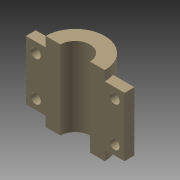
# Autodesk Inventor part: 砂轮架带动曲柄轴盖
Saved by Autodesk Inventor 2015 (Build 190159000, 159)
## iProperties
Created: 2017-05-17
Part Number: 砂轮架带动曲柄轴盖
Material: 常规
Document SubType Name: Modeling
Designer: Administrator
Density: 1 g/cm^3
Appearance: 麦色
Author: Administrator
Autodesk Inventor part; units mm, degrees
ref_plane "YZ Plane" through (0, 0, 0) normal (1, 0, 0) x (0, 1, 0)
ref_plane "XZ Plane" through (0, 0, 0) normal (0, 1, 0) x (-1, 0, 0)
ref_plane "XY Plane" through (0, 0, 0) normal (0, 0, 1) x (1, 0, 0)
sketch "草图1" plane through (0, 0, 0) normal (0, 0, 1) x (1, 0, 0)
  arc A0 (7.5, 0) -> (-7.5, 0) centre (0, 0) ccw
  arc A1 (15, 0) -> (-15, 0) centre (0, 0) ccw
  line L0 (25, 5) -> (25, 0)
  line L1 (-25, 0) -> (-25, 5)
  line L2 (25, 0) -> (7.5, 0)
  line L3 (-7.5, 0) -> (-25, 0)
  line L4 (-25, 5) -> (-5.5902, 5)
  line L5 (5.5902, 5) -> (25, 5)
  line L6 (0, 0) -> (0, -4.0409)
  line L7 (0, 0) -> (2.0046, 0)
  arc A2 (5.5902, 5) -> (-5.5902, 5) centre (0, 0) ccw
  arc A3 (14.1421, 5) -> (-14.1421, 5) centre (0, 0) ccw
  dimension "d0" = 15
  dimension "d1" = 30
  dimension "d2" = 5
  dimension "d3" = 50
  dimension "d4" = 4.0409
  dimension "d5" = 2.0046
  constraints: 16 end point, 12 point on circle, 5 parallel, 4 centre point, 4 point on line, 3 coincident, 3 collinear, 3 horizontal, 2 concentric, 2 perpendicular, 1 vertical, 1 other
  measures "d0" diameter of A0
  measures "d1" diameter of A1
  measures "d2" distance of L0.start L0.end
  measures "d3" distance of L1.end L0.start
  measures "d4" distance of L6.start L6.end
  measures "d5" distance of L6.start L7.end
extrude "拉伸1" add sketch "草图1" along normal blind 40
sketch "草图2" plane through (0, 0, 40) normal (0, 0, 1) x (1, 0, 0)
  line L0 (14.1421, 5) -> (25, 5)
  line L1 (25, 5) -> (14.1421, 5) projected
  line L2 (25, 5) -> (25, 0)
  line L3 (25, 0) -> (15, 0)
  line L4 (7.5, 0) -> (25, 0) projected
  line L5 (-14.1421, 5) -> (-25, 5)
  line L6 (-14.1421, 5) -> (-25, 5) projected
  line L7 (-25, 5) -> (-25, 0)
  line L8 (-25, 0) -> (-15, 0)
  arc A0 (15, 0) -> (14.1421, 5) centre (0, 0) ccw
  arc A1 (-14.1421, 5) -> (-15, 0) centre (0, 0) ccw
  constraints: 12 end point, 4 point on circle, 3 collinear, 3 perpendicular, 2 centre point, 2 coincident, 1 point on line
extrude "拉伸2" cut sketch "草图2" against normal blind 5
pattern_linear "矩形阵列1" count 2 spacing 35 along (0, 0, -1) of "拉伸2"
fillet "圆角1" radius 0.25 2 edges at (14.1421, 5, 20) (-14.1421, 5, 20)
sketch "草图3" plane through (25, 5, 35) normal (0, 1, 0) x (1, 0, 0)
  circle A0 centre (-5, 25) radius 2.5
  circle A1 centre (-5, 5) radius 2.5
  circle A2 centre (-45, 25) radius 2.5
  circle A3 centre (-45, 5) radius 2.5
  line L0 (0, 30) -> (0, 0) projected
  line L1 (0, 30) -> (-10.6822, 30) projected
  line L2 (-10.6822, 0) -> (0, 0) projected
  line L3 (-50, 30) -> (-50, 0) projected
  line L4 (-50, 0) -> (-39.3178, 0) projected
  line L5 (-39.3178, 30) -> (-50, 30) projected
  point P0 (-25, 35)
  dimension "d14" = 5
  dimension "d15" = 5
  dimension "d16" = 5
  dimension "d17" = 5
  dimension "d18" = 5
  dimension "d19" = 5
  dimension "d20" = 5
  dimension "d21" = 5
  dimension "d22" = 5
  dimension "d23" = 5
  dimension "d24" = 5
  dimension "d25" = 5
  constraints: 4 centre point
  measures "d14" diameter of A0
  measures "d15" diameter of A1
  measures "d16" diameter of A2
  measures "d17" diameter of A3
  measures "d18" distance from line of L0 A0.centre
  measures "d19" distance from line of A0.centre L1
  measures "d20" distance from line of A1.centre L2
  measures "d21" distance from line of A1.centre L0
  measures "d22" distance from line of A3.centre L3
  measures "d23" distance from line of A3.centre L4
  measures "d24" distance from line of L5 A2.centre
  measures "d25" distance from line of A2.centre L3
extrude "拉伸3" cut sketch "草图3" against normal through all
